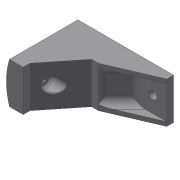
# Autodesk Inventor part: Switch_Panel
Saved by Autodesk Inventor 2018 (Build 220112000, 112)
## iProperties
Created: 2019-11-23
Part Number: Switch_Panel
Material: Generic
Document SubType Name: Modeling
Designer: Clevo
Density: 1 g/cm^3
Appearance: Default
Author: Clevo
Autodesk Inventor part; units mm, degrees
ref_plane "YZ Plane" through (0, 0, 0) normal (1, 0, 0) x (0, 1, 0)
ref_plane "XZ Plane" through (0, 0, 0) normal (0, 1, 0) x (-1, 0, 0)
ref_plane "XY Plane" through (0, 0, 0) normal (0, 0, 1) x (1, 0, 0)
sketch "Sketch1" plane through (0, 0, 0) normal (0, 1, 0) x (-1, 0, 0)
  circle A0 centre (0, 0) radius 50
  line L0 (47.697, 15) -> (-22.303, 15)
  line L1 (-22.303, 15) -> (-22.303, -15)
  line L2 (-22.303, -15) -> (47.697, -15)
  line L3 (47.697, -15) -> (47.697, 15)
  dimension "d0" = 100
  dimension "d1" = 30
  dimension "d4" = 70
  constraints: 8 end point, 2 parallel, 2 point on circle, 1 centre point, 1 horizontal, 1 perpendicular
  measures "d0" diameter of A0
  measures "d1" distance of L0.end L1.end
  measures "d4" distance of L1.end L2.end
extrude "Extrusion1" add sketch "Sketch1" along normal blind 50 contours A0 L3 | L3 L2 L1 L0
sketch "Sketch2" plane through (0, 0, 0) normal (0, -1, 0) x (1, 0, 0)
  arc A0 (-47.697, 15) -> (-47.697, -15) centre (0, 0) ccw projected
  line L0 (22.303, -15) -> (-47.697, -15) projected
  line L1 (22.303, 15) -> (22.303, -15) projected
  line L2 (-47.697, 15) -> (22.303, 15) projected
  line L3 (22.303, 15) -> (22.303, -15) projected
  line L4 (22.303, -15) -> (-47.697, -15) projected
  line L5 (22.303, 15) -> (-37.697, 15)
  line L6 (-37.697, 15) -> (-37.697, -15)
  line L7 (-37.697, -15) -> (22.303, -15)
  line L8 (22.303, -15) -> (22.303, 15)
  dimension "d5" = 60
  constraints: 8 end point, 2 parallel, 1 horizontal, 1 perpendicular, 1 point on line
  measures "d5" distance between parallel lines of L1 L6
extrude "Extrusion2" cut sketch "Sketch2" against normal blind 30 contours L2 L1 L0 L6
sketch "Sketch3" plane through (0, 30, 0) normal (0, -1, 0) x (1, 0, 0)
  line L0 (22.303, -15) -> (-37.697, -15) projected
  line L1 (22.303, 15) -> (22.303, -15) projected
  line L2 (-37.697, 15) -> (22.303, 15) projected
  line L3 (-37.697, -15) -> (-37.697, 15) projected
  line L4 (-47.697, 15) -> (22.303, 15) projected
  line L5 (22.303, -15) -> (-47.697, -15) projected
  line L6 (22.303, 15) -> (-12.697, 15)
  line L7 (-12.697, 15) -> (-12.697, -15)
  line L8 (-12.697, -15) -> (22.303, -15)
  line L9 (22.303, -15) -> (22.303, 15)
  point P0 (0, 0)
  dimension "d8" = 35
  constraints: 8 end point, 2 parallel, 1 horizontal, 1 midpoint, 1 perpendicular
  measures "d8" distance between parallel lines of L1 L7
extrude "Extrusion3" cut sketch "Sketch3" against normal blind 15 contours L0 L7 L2 L1
sketch "Sketch4" plane through (0, 45, 0) normal (0, -1, 0) x (1, 0, 0)
  point P0 (0, 0)
  point P1 (12, 0)
  dimension "d11" = 12
  constraints: 1 horizontal alignment
  measures "d11" distance of point (0, 0) point (12, 0)
hole "Hole1" at (12, 45, 0) direction (0, 1, 0) diameter 6 end through all
sketch "Sketch5" plane through (-47.697, 50, 15) normal (0, 0, 1) x (1, 0, 0)
  line L0 (35, -5) -> (70, -5) projected
  line L1 (70, -5) -> (70, 0) projected
  line L2 (0, 0) -> (70, 0) projected
  line L3 (0, -50) -> (0, 0) projected
  line L4 (0, -50) -> (10, -50) projected
  line L5 (10, -50) -> (10, -20) projected
  line L6 (10, -20) -> (35, -20) projected
  line L7 (35, -20) -> (35, -5) projected
  line L8 (35, -20) -> (35, -5) projected
  line L9 (35, -20) -> (70, -5)
  point P0 (47.697, -50)
  constraints: 2 end point
extrude "Extrusion4" add sketch "Sketch5" against normal blind 3 contours L0 L9 L7
mirror "Mirror1" about plane through (0, 0, 0) normal (0, 0, 1) of "Extrusion4"
chamfer "Chamfer1" distance 12 angle 45 1 edges at (-12.697, 45, 0)
fillet "Fillet1" radius 5 4 edges at (-12.697, 33, 0) (-6.697, 39, 12) (-6.697, 39, -12) (-0.697, 45, 0)
chamfer "Chamfer2" distance 25 distance2 20 1 edges at (-37.697, 30, 0) measured on face at (-37.697, 29.5, 0)
sketch "Sketch6" plane through (22.303, 50, 15) normal (1, 0, 0) x (0, 0, -1)
  line L0 (0, -5) -> (3, -5) projected
  line L1 (3, -5) -> (27, -5) projected
  line L2 (27, -5) -> (30, -5) projected
  line L3 (30, -5) -> (30, 0) projected
  line L4 (0, 0) -> (30, 0) projected
  line L5 (0, -5) -> (0, 0) projected
  circle A0 centre (15, -35) radius 5
  point P0 (15, -50)
  dimension "d28" = 15
  dimension "d29" = 10
  constraints: 1 centre point, 1 vertical alignment
  measures "d28" distance of point (15, -50) A0.centre
  measures "d29" diameter of A0
extrude "Extrusion5" cut sketch "Sketch6" against normal blind 60 contours A0
fillet "Fillet2" radius 0.5 1 edges at (-29.697, 15, 5)
fillet "Fillet3" radius 2 1 edges at (-37.697, 15, 5)
sketch "Sketch7" plane through (-37.697, 15, 0) normal (1, 0, 0) x (0, 0, -1)
  circle A0 centre (0, 0) radius 3 projected
  point P0 (0, -15)
hole "Hole2" at (-37.697, 15, 0) direction (-1, 0, 0) diameter 4.3 end through all clearance for "Flat Head Machine Screw" size "M4" standard "Ansi Metric M Profile"
body "Solid1"
